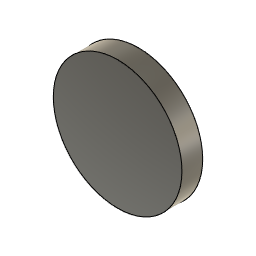
diaphragm_stencil v3 (Autodesk Fusion 360 design; units mm, degrees)
Autodesk Fusion 360 part; units mm, degrees
sketch "62mm" plane through (0, 0, 0) normal (0, 1, 0) x (1, 0, 0)
  circle A0 centre (0, -25) radius 31
  dimension "d1" = 62
  measures "d1" diameter of A0
extrude "Extrude1" add sketch "62mm" along normal blind 10
named bodies: "stencil"
